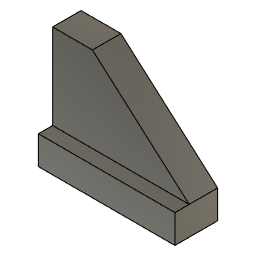
Attic Wardrobe (Autodesk Fusion 360 design; units mm, degrees)
Autodesk Fusion 360 part; units mm, degrees
sketch "Sketch1" plane through (0, 0, 0) normal (0, 1, 0) x (1, 0, 0)
  line L0 (0, 0) -> (2400, 0)
  line L1 (0, 0) -> (0, -2000)
  line L2 (0, -2000) -> (700, -2000)
  line L3 (2400, 0) -> (2400, -500)
  line L4 (700, -2000) -> (2400, -500)
  dimension "d1" = 2400
  dimension "d2" = 2000
  dimension "d3" = 700
  dimension "d4" = 500
  constraint coincident L0.start L1.start
  constraint horizontal L0
  constraint perpendicular L0 L1
  constraint perpendicular L1 L2
  constraint perpendicular L0 L3
  measures "d1" distance of L0.start L0.end
  measures "d2" distance of L0.start L1.end
  measures "d3" distance of L1.end L2.end
  measures "d4" distance of L0.end L3.end
extrude "Extrude1" add sketch "Sketch1" along normal blind 500 makes body 1
move_face "OffsetFaces1" offset -500 1 faces at (800, 166.6667, 0) on bodies 1
sketch "Sketch2" plane through (0, 0, 0) normal (-1, 0, 0) x (0, -1, 0)
  line L0 (0, 500) -> (0, 2000)
  line L1 (0, 2000) -> (-500, 2000)
  line L2 (-500, 2000) -> (-500, 500)
  line L3 (-500, 500) -> (0, 500)
  line L4 (-500, 500) -> (250, 500)
  line L5 (250, 500) -> (250, 0)
  line L6 (250, 0) -> (-500, 0)
  line L7 (-500, 0) -> (-500, 500)
  dimension "d8" = 750
  constraint horizontal L4
  constraint vertical L5
  constraint horizontal L6
  constraint vertical L7
  constraint coincident L2.end L3.start
  constraint coincident origin L6
  measures "d8" distance of L5 L7
extrude "Extrude2" add sketch "Sketch2" against normal blind 2400 separate body contours L3 L4 L5 L6 L7 makes body 2
named bodies: "Top", "Bottom"
